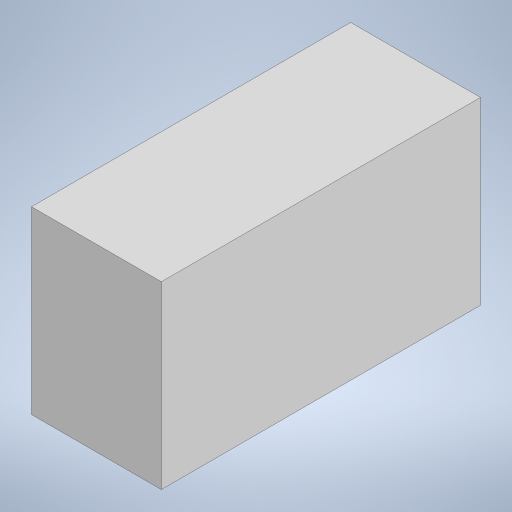
# Autodesk Inventor part: JST4-m
Saved by Autodesk Inventor 2023.4 (Build 274418000, 418)
## iProperties
Created: 2023-09-18
Part Number: JST4-m
Material: Generic
Document SubType Name: Modeling
Designer: shpctac10021
Density: 1 g/cm^3
Appearance: Default
Author: shpctac10021
Autodesk Inventor part; units mm, degrees
ref_plane "YZ Plane" through (0, 0, 0) normal (1, 0, 0) x (0, 1, 0)
ref_plane "XZ Plane" through (0, 0, 0) normal (0, 1, 0) x (-1, 0, 0)
ref_plane "XY Plane" through (0, 0, 0) normal (0, 0, 1) x (1, 0, 0)
sketch "Sketch1" plane through (0, 0, 0) normal (0, 1, 0) x (-1, 0, 0)
  line L0 (0, 0) -> (3.5, 0)
  line L1 (3.5, 0) -> (3.5, -8.6)
  line L2 (3.5, -8.6) -> (0, -8.6)
  line L3 (0, -8.6) -> (0, 0)
  dimension "d0" = 3.5
  dimension "d1" = 8.6
  constraints: 8 end point, 2 parallel, 1 horizontal, 1 perpendicular
  measures "d0" distance of L0.start L0.end
  measures "d1" distance of L0.end L1.end
extrude "Extrusion1" add sketch "Sketch1" along normal blind 4.85
body "Solid1"
